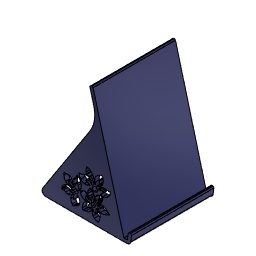
Portafoto (Autodesk Fusion 360 design; units mm, degrees)
Autodesk Fusion 360 part; units mm, degrees
sketch "Schizzo1" plane through (0, 0, 0) normal (0, 1, 0) x (1, 0, 0)
  line L0 (0, 0) -> (131.7113, 0) construction
  line L1 (79.5451, 0) -> (58.8396, -77.2741)
  line L2 (79.5451, 0) -> (81.9451, 0)
  line L3 (81.9451, 0) -> (82.641, -4.9513)
  line L4 (77.857, 2.2) -> (56.7146, -76.7047)
  line L5 (77.857, 2.2) -> (83.8576, 2.2)
  line L6 (83.8576, 2.2) -> (84.8196, -4.6452)
  line L7 (82.641, -4.9513) -> (84.8196, -4.6452)
  line L8 (77.857, 2.2) -> (22.857, 2.2)
  line L9 (22.857, 2.2) -> (61.7467, -57.9244)
  line L10 (56.7146, -76.7047) -> (58.8396, -77.2741)
  dimension "d1" = 75
  dimension "d2" = 2.4
  dimension "d3" = 5
  dimension "d4" = 80
  dimension "d5" = 2.2
  dimension "d6" = 55
  dimension "d23" = 98
  constraint coincident L0.start origin
  constraint horizontal L0
  constraint coincident L0 L1.start
  constraint coincident L0 L2.end
  constraint parallel L5 L8
  constraint coincident L4 L9.end
  measures "d1" angle of L0 L1
  measures "d2" distance of L1.start L2.end
  measures "d3" distance of L2.end L3.end
  measures "d4" distance of L1.start L1.end
  measures "d6" distance of L4.start L8.end
  measures "d23" angle of L2 L3
extrude "Estrusione1" add sketch "Schizzo1" along normal blind 55 contours L1 L2 L3 L4 L5 L6 L7 L10
extrude "Estrusione2" add sketch "Schizzo1" along normal blind 3 contours L4 L8 L9
fillet "Raccordo1" radius 2.5 1 edges at (83.8576, 27.5, -2.2)
fillet "Raccordo3" radius 0.75 2 edges at (82.641, 27.5, 4.9513) (84.8196, 27.5, 4.6452)
fillet "Raccordo4" radius 0.75 2 edges at (58.8396, 27.5, 77.2741) (56.7146, 27.5, 76.7047)
fillet "Raccordo5" radius 20 1 edges at (61.7467, 1.5, 57.9244)
fillet "Raccordo6" radius 2.5 1 edges at (22.857, 1.5, -2.2)
sketch "Schizzo3" plane through (0, 0, 0) normal (0, -1, 0) x (1, 0, 0)
  arc A0 (25.3523, 1.6578) -> (27.4515, -2.2) centre (27.4515, 0.3) ccw
  line L0 (27.4515, -2.2) -> (81.6844, -2.2)
  arc A1 (81.6844, -2.2) -> (84.16, -0.0479) centre (81.6844, 0.3) ccw
  line L1 (84.16, -0.0479) -> (84.7152, 3.9025)
  arc A2 (84.7152, 3.9025) -> (84.0769, 4.7495) centre (83.9725, 4.0068) ccw
  line L2 (84.0769, 4.7495) -> (83.3837, 4.847)
  arc A3 (83.3837, 4.847) -> (82.5366, 4.2086) centre (83.2793, 4.1043) ccw
  line L3 (82.5366, 4.2086) -> (81.9451, 0)
  line L4 (81.9451, 0) -> (79.5451, 0)
  line L5 (79.5451, 0) -> (59.0337, 76.5496)
  arc A4 (59.0337, 76.5496) -> (58.1152, 77.08) centre (58.3093, 76.3555) ccw
  line L6 (58.1152, 77.08) -> (57.439, 76.8988)
  arc A5 (57.439, 76.8988) -> (56.9087, 75.9802) centre (57.6331, 76.1743) ccw
  line L7 (56.9087, 75.9802) -> (59.4477, 66.5045)
  arc A6 (56.9224, 50.4659) -> (59.4477, 66.5045) centre (40.1292, 61.3281) ccw
  line L8 (56.9224, 50.4659) -> (25.3523, 1.6578)
  spline S0 degree 3 poles (64.7057, 28.6744) (64.5776, 28.5377) (64.293, 28.3413) (64.088, 28.2503) knots 0 0 0 0 1 1 1 1
  spline S1 degree 3 poles (64.088, 28.2503) (63.9912, 28.2076) (63.7037, 28.1022) (63.4533, 28.0197) knots 0 0 0 0 1 1 1 1
  spline S2 degree 3 poles (63.4533, 28.0197) (62.9096, 27.8432) (62.1667, 27.4931) (61.8422, 27.2625) knots 0 0 0 0 1 1 1 1
  spline S3 degree 3 poles (61.8422, 27.2625) (61.3212, 26.8953) (60.9512, 26.4627) (60.6609, 25.8706) knots 0 0 0 0 1 1 1 1
  spline S4 degree 3 poles (60.6609, 25.8706) (60.1001, 24.7377) (60.0005, 23.6077) (60.3392, 22.2271) knots 0 0 0 0 1 1 1 1
  spline S5 degree 3 poles (60.3392, 22.2271) (60.4104, 21.9453) (60.5897, 21.3817) (60.6239, 21.3476) knots 0 0 0 0 1 1 1 1
  spline S6 degree 3 poles (60.6239, 21.3476) (60.6381, 21.3305) (60.6495, 21.3874) (60.6495, 21.4785) knots 0 0 0 0 1 1 1 1
  spline S7 degree 3 poles (60.6495, 21.4785) (60.6495, 21.5696) (60.6694, 21.7859) (60.6922, 21.9624) knots 0 0 0 0 1 1 1 1
  spline S8 degree 3 poles (60.6922, 21.9624) (60.8317, 23.027) (61.2985, 23.8268) (62.0499, 24.288) knots 0 0 0 0 1 1 1 1
  spline S9 degree 3 poles (62.0499, 24.288) (62.3061, 24.4474) (62.7701, 24.6125) (62.9181, 24.5982) knots 0 0 0 0 1 1 1 1
  spline S10 degree 3 poles (62.9181, 24.5982) (63.0092, 24.5897) (63.0263, 24.5755) (63.0576, 24.4815) knots 0 0 0 0 1 1 1 1
  spline S11 degree 3 poles (63.0576, 24.4815) (63.2085, 24.0432) (63.1658, 23.3287) (62.9494, 22.7309) knots 0 0 0 0 1 1 1 1
  spline S12 degree 3 poles (62.9494, 22.7309) (62.7957, 22.3068) (62.6306, 22.1019) (61.808, 21.302) knots 0 0 0 0 1 1 1 1
  spline S13 degree 3 poles (61.808, 21.302) (61.5205, 21.0259) (61.3412, 20.7868) (61.2899, 20.6217) knots 0 0 0 0 1 1 1 1
  spline S14 degree 3 poles (61.2899, 20.6217) (61.27, 20.5591) (61.2757, 20.5562) (61.3497, 20.5733) knots 0 0 0 0 1 1 1 1
  spline S15 degree 3 poles (61.3497, 20.5733) (61.5461, 20.6189) (61.9987, 20.7783) (62.3004, 20.9092) knots 0 0 0 0 1 1 1 1
  spline S16 degree 3 poles (62.3004, 20.9092) (63.6354, 21.4813) (64.7142, 22.4121) (65.2579, 23.4653) knots 0 0 0 0 1 1 1 1
  spline S17 degree 3 poles (65.2579, 23.4653) (65.645, 24.2168) (65.8187, 25.0594) (65.7931, 26.0414) knots 0 0 0 0 1 1 1 1
  spline S18 degree 3 poles (65.7931, 26.0414) (65.776, 26.6135) (65.7304, 26.9039) (65.5853, 27.3735) knots 0 0 0 0 1 1 1 1
  spline S19 degree 3 poles (65.5853, 27.3735) (65.4515, 27.8005) (65.1498, 28.3556) (64.885, 28.6545) knots 0 0 0 0 1 1 1 1
  line L9 (64.885, 28.6545) -> (64.7911, 28.7655)
  line L10 (64.7911, 28.7655) -> (64.7057, 28.6744)
  spline S20 degree 3 poles (54.6121, 28.7114) (54.6093, 28.7) (54.6093, 28.6772) (54.6121, 28.663) knots 0 0 0 0 1 1 1 1
  spline S21 degree 3 poles (54.6121, 28.663) (54.6263, 28.5947) (54.5466, 27.9428) (54.4584, 27.4077) knots 0 0 0 0 1 1 1 1
  spline S22 degree 3 poles (54.4584, 27.4077) (54.3161, 26.5538) (54.2734, 26.1325) (54.2734, 25.6287) knots 0 0 0 0 1 1 1 1
  spline S23 degree 3 poles (54.2734, 25.6287) (54.2734, 25.1419) (54.3246, 24.7605) (54.4242, 24.4644) knots 0 0 0 0 1 1 1 1
  line L11 (54.4242, 24.4644) -> (54.4897, 24.2766)
  line L12 (54.4897, 24.2766) -> (54.8284, 24.2567)
  spline S24 degree 3 poles (54.8284, 24.2567) (55.3778, 24.2253) (55.8304, 24.0802) (56.2631, 23.7955) knots 0 0 0 0 1 1 1 1
  line L13 (56.2631, 23.7955) -> (56.4908, 23.6447)
  line L14 (56.4908, 23.6447) -> (56.5392, 23.8012)
  spline S25 degree 3 poles (56.5392, 23.8012) (56.5619, 23.8895) (56.6217, 24.0147) (56.6701, 24.0802) knots 0 0 0 0 1 1 1 1
  spline S26 degree 3 poles (56.6701, 24.0802) (56.7783, 24.2339) (57.043, 24.4616) (57.1113, 24.4616) knots 0 0 0 0 1 1 1 1
  spline S27 degree 3 poles (57.1113, 24.4616) (57.1398, 24.4616) (57.2508, 24.4303) (57.359, 24.3904) knots 0 0 0 0 1 1 1 1
  spline S28 degree 3 poles (57.359, 24.3904) (58.1901, 24.0972) (58.9331, 22.99) (59.4113, 21.3305) knots 0 0 0 0 1 1 1 1
  spline S29 degree 3 poles (59.4113, 21.3305) (59.4625, 21.1483) (59.5137, 20.9547) (59.5251, 20.895) knots 0 0 0 0 1 1 1 1
  spline S30 degree 3 poles (59.5251, 20.895) (59.5536, 20.7413) (59.5821, 20.7441) (59.6333, 20.912) knots 0 0 0 0 1 1 1 1
  spline S31 degree 3 poles (59.6333, 20.912) (59.9635, 21.9595) (59.8325, 23.6048) (59.3173, 24.917) knots 0 0 0 0 1 1 1 1
  spline S32 degree 3 poles (59.3173, 24.917) (58.8761, 26.0442) (58.3353, 26.827) (57.5127, 27.5386) knots 0 0 0 0 1 1 1 1
  spline S33 degree 3 poles (57.5127, 27.5386) (56.8437, 28.1136) (55.9101, 28.5377) (55.0135, 28.6715) knots 0 0 0 0 1 1 1 1
  spline S34 degree 3 poles (55.0135, 28.6715) (54.8968, 28.6915) (54.7573, 28.7114) (54.7089, 28.7199) knots 0 0 0 0 1 1 1 1
  spline S35 degree 3 poles (54.7089, 28.7199) (54.6577, 28.7285) (54.6121, 28.7228) (54.6121, 28.7114) knots 0 0 0 0 1 1 1 1
  spline S36 degree 3 poles (54.1026, 23.7614) (53.5646, 23.6874) (53.1206, 23.545) (52.2524, 23.1608) knots 0 0 0 0 1 1 1 1
  spline S37 degree 3 poles (52.2524, 23.1608) (51.333, 22.7537) (51.0284, 22.6569) (50.5018, 22.6114) knots 0 0 0 0 1 1 1 1
  spline S38 degree 3 poles (50.5018, 22.6114) (50.2314, 22.5886) (49.8073, 22.6085) (49.6165, 22.6569) knots 0 0 0 0 1 1 1 1
  spline S39 degree 3 poles (49.6165, 22.6569) (49.5482, 22.674) (49.5482, 22.6712) (49.5482, 22.489) knots 0 0 0 0 1 1 1 1
  spline S40 degree 3 poles (49.5482, 22.489) (49.5482, 21.7005) (50.035, 20.5648) (50.7324, 19.7393) knots 0 0 0 0 1 1 1 1
  spline S41 degree 3 poles (50.7324, 19.7393) (51.4326, 18.9024) (52.1755, 18.4385) (53.112, 18.2449) knots 0 0 0 0 1 1 1 1
  spline S42 degree 3 poles (53.112, 18.2449) (53.9375, 18.0741) (54.5409, 18.1424) (55.4604, 18.5096) knots 0 0 0 0 1 1 1 1
  spline S43 degree 3 poles (55.4604, 18.5096) (56.1094, 18.7687) (56.2204, 18.8) (56.5449, 18.817) knots 0 0 0 0 1 1 1 1
  spline S44 degree 3 poles (56.5449, 18.817) (56.8779, 18.837) (56.8807, 18.837) (56.764, 19.0732) knots 0 0 0 0 1 1 1 1
  spline S45 degree 3 poles (56.764, 19.0732) (56.5534, 19.4945) (55.9386, 19.8959) (55.1643, 20.1179) knots 0 0 0 0 1 1 1 1
  spline S46 degree 3 poles (55.1643, 20.1179) (54.8, 20.2232) (54.3189, 20.3057) (54.0741, 20.3057) knots 0 0 0 0 1 1 1 1
  spline S47 degree 3 poles (54.0741, 20.3057) (53.9261, 20.3057) (53.9261, 20.3057) (53.9432, 20.3854) knots 0 0 0 0 1 1 1 1
  spline S48 degree 3 poles (53.9432, 20.3854) (53.9546, 20.4281) (54.0087, 20.5278) (54.0627, 20.6075) knots 0 0 0 0 1 1 1 1
  spline S49 degree 3 poles (54.0627, 20.6075) (54.336, 21.0088) (54.9309, 21.2906) (55.6682, 21.3646) knots 0 0 0 0 1 1 1 1
  spline S50 degree 3 poles (55.6682, 21.3646) (55.9585, 21.3931) (56.0297, 21.3903) (56.2517, 21.3476) knots 0 0 0 0 1 1 1 1
  spline S51 degree 3 poles (56.2517, 21.3476) (56.7783, 21.2422) (57.1227, 21.0629) (57.5212, 20.6843) knots 0 0 0 0 1 1 1 1
  spline S52 degree 3 poles (57.5212, 20.6843) (57.7375, 20.4765) (58.099, 20.0382) (58.2186, 19.8332) knots 0 0 0 0 1 1 1 1
  spline S53 degree 3 poles (58.2186, 19.8332) (58.2812, 19.7308) (58.3011, 19.8275) (58.2983, 20.1862) knots 0 0 0 0 1 1 1 1
  spline S54 degree 3 poles (58.2983, 20.1862) (58.2954, 20.5875) (58.23, 20.9377) (58.082, 21.3561) knots 0 0 0 0 1 1 1 1
  spline S55 degree 3 poles (58.082, 21.3561) (57.6521, 22.5772) (56.6559, 23.4539) (55.412, 23.7073) knots 0 0 0 0 1 1 1 1
  spline S56 degree 3 poles (55.412, 23.7073) (55.2013, 23.7528) (54.3047, 23.787) (54.1026, 23.7614) knots 0 0 0 0 1 1 1 1
  spline S57 degree 3 poles (65.8443, 22.1673) (65.7988, 22.1616) (65.6621, 22.1417) (65.5454, 22.1246) knots 0 0 0 0 1 1 1 1
  spline S58 degree 3 poles (65.5454, 22.1246) (65.0444, 22.0563) (64.3328, 21.7574) (63.9201, 21.4472) knots 0 0 0 0 1 1 1 1
  spline S59 degree 3 poles (63.9201, 21.4472) (63.5273, 21.1483) (63.0918, 20.6132) (62.9124, 20.209) knots 0 0 0 0 1 1 1 1
  spline S60 degree 3 poles (62.9124, 20.209) (62.8185, 19.9983) (62.7103, 19.6482) (62.6676, 19.4319) knots 0 0 0 0 1 1 1 1
  spline S61 degree 3 poles (62.6676, 19.4319) (62.6392, 19.2839) (62.642, 19.2355) (62.6847, 19.1045) knots 0 0 0 0 1 1 1 1
  spline S62 degree 3 poles (62.6847, 19.1045) (62.7559, 18.891) (62.7559, 18.891) (62.8413, 19.0277) knots 0 0 0 0 1 1 1 1
  spline S63 degree 3 poles (62.8413, 19.0277) (62.9523, 19.2042) (63.1743, 19.4205) (63.3622, 19.5344) knots 0 0 0 0 1 1 1 1
  spline S64 degree 3 poles (63.3622, 19.5344) (63.7208, 19.7478) (64.3072, 19.8759) (64.7484, 19.8389) knots 0 0 0 0 1 1 1 1
  spline S65 degree 3 poles (64.7484, 19.8389) (64.9647, 19.819) (65.4031, 19.7251) (65.497, 19.6767) knots 0 0 0 0 1 1 1 1
  spline S66 degree 3 poles (65.497, 19.6767) (65.5995, 19.6197) (65.5113, 19.1472) (65.3291, 18.7857) knots 0 0 0 0 1 1 1 1
  spline S67 degree 3 poles (65.3291, 18.7857) (65.0444, 18.2278) (64.4552, 17.6187) (63.9002, 17.3113) knots 0 0 0 0 1 1 1 1
  line L15 (63.9002, 17.3113) -> (63.7237, 17.2116)
  line L16 (63.7237, 17.2116) -> (63.9571, 17.1376)
  spline S68 degree 3 poles (63.9571, 17.1376) (64.5805, 16.9412) (64.9533, 16.8843) (65.5739, 16.8843) knots 0 0 0 0 1 1 1 1
  spline S69 degree 3 poles (65.5739, 16.8843) (66.3396, 16.8871) (66.9459, 17.0323) (67.666, 17.391) knots 0 0 0 0 1 1 1 1
  spline S70 degree 3 poles (67.666, 17.391) (68.1357, 17.6215) (68.4887, 17.8749) (68.9014, 18.2705) knots 0 0 0 0 1 1 1 1
  spline S71 degree 3 poles (68.9014, 18.2705) (69.6557, 18.9992) (70.1681, 19.8617) (70.373, 20.7555) knots 0 0 0 0 1 1 1 1
  spline S72 degree 3 poles (70.373, 20.7555) (70.447, 21.0828) (70.4897, 21.6322) (70.4584, 21.8485) knots 0 0 0 0 1 1 1 1
  line L17 (70.4584, 21.8485) -> (70.4385, 21.9795)
  line L18 (70.4385, 21.9795) -> (70.3161, 21.9282)
  spline S73 degree 3 poles (70.3161, 21.9282) (70.0058, 21.7888) (69.4622, 21.8001) (68.2866, 21.9681) knots 0 0 0 0 1 1 1 1
  spline S74 degree 3 poles (68.2866, 21.9681) (67.9137, 22.0222) (67.4355, 22.0876) (67.2248, 22.1104) knots 0 0 0 0 1 1 1 1
  spline S75 degree 3 poles (67.2248, 22.1104) (66.8349, 22.156) (66.0009, 22.1901) (65.8443, 22.1673) knots 0 0 0 0 1 1 1 1
  spline S76 degree 3 poles (48.2844, 20.7099) (48.2759, 20.7014) (48.2673, 20.6502) (48.2673, 20.5932) knots 0 0 0 0 1 1 1 1
  spline S77 degree 3 poles (48.2673, 20.5932) (48.2673, 20.3655) (48.0937, 19.9841) (47.8233, 19.6027) knots 0 0 0 0 1 1 1 1
  spline S78 degree 3 poles (47.8233, 19.6027) (47.7293, 19.4746) (47.4561, 19.1387) (47.2141, 18.854) knots 0 0 0 0 1 1 1 1
  spline S79 degree 3 poles (47.2141, 18.854) (46.2805, 17.7582) (45.9218, 17.2059) (45.6913, 16.5114) knots 0 0 0 0 1 1 1 1
  spline S80 degree 3 poles (45.6913, 16.5114) (45.4066, 15.6432) (45.4493, 14.5587) (45.7994, 13.8443) knots 0 0 0 0 1 1 1 1
  spline S81 degree 3 poles (45.7994, 13.8443) (45.9617, 13.5084) (46.3061, 13.1611) (46.6221, 13.0102) knots 0 0 0 0 1 1 1 1
  spline S82 degree 3 poles (46.6221, 13.0102) (46.7445, 12.9505) (46.8839, 12.8964) (46.9323, 12.885) knots 0 0 0 0 1 1 1 1
  line L19 (46.9323, 12.885) -> (47.0206, 12.8679)
  line L20 (47.0206, 12.8679) -> (46.9949, 13.0074)
  spline S83 degree 3 poles (46.9949, 13.0074) (46.9551, 13.2436) (46.9722, 13.8955) (47.0234, 14.1061) knots 0 0 0 0 1 1 1 1
  spline S84 degree 3 poles (47.0234, 14.1061) (47.1003, 14.4135) (47.234, 14.7352) (47.3906, 14.9743) knots 0 0 0 0 1 1 1 1
  spline S85 degree 3 poles (47.3906, 14.9743) (47.5699, 15.2504) (47.9684, 15.6489) (48.2018, 15.7912) knots 0 0 0 0 1 1 1 1
  line L21 (48.2018, 15.7912) -> (48.3812, 15.8966)
  line L22 (48.3812, 15.8966) -> (48.4979, 15.8026)
  spline S86 degree 3 poles (48.4979, 15.8026) (48.6459, 15.6831) (48.8452, 15.4184) (48.9647, 15.1821) knots 0 0 0 0 1 1 1 1
  spline S87 degree 3 poles (48.9647, 15.1821) (49.2636, 14.5843) (49.386, 13.9012) (49.3888, 12.8138) knots 0 0 0 0 1 1 1 1
  line L23 (49.3888, 12.8138) -> (49.3888, 12.199)
  line L24 (49.3888, 12.199) -> (49.5454, 12.2986)
  spline S88 degree 3 poles (49.5454, 12.2986) (50.2912, 12.7711) (50.7836, 13.4714) (51.0142, 14.3822) knots 0 0 0 0 1 1 1 1
  spline S89 degree 3 poles (51.0142, 14.3822) (51.2277, 15.2305) (51.2163, 16.3292) (50.9857, 17.3027) knots 0 0 0 0 1 1 1 1
  spline S90 degree 3 poles (50.9857, 17.3027) (50.6612, 18.669) (49.867, 19.8218) (48.8081, 20.468) knots 0 0 0 0 1 1 1 1
  spline S91 degree 3 poles (48.8081, 20.468) (48.5833, 20.6046) (48.3072, 20.7327) (48.2844, 20.7099) knots 0 0 0 0 1 1 1 1
  spline S92 degree 3 poles (59.9521, 20.0809) (59.1038, 19.9414) (58.5146, 19.2981) (58.5146, 18.5125) knots 0 0 0 0 1 1 1 1
  spline S93 degree 3 poles (58.5146, 18.5125) (58.5146, 17.8179) (58.9786, 17.2287) (59.7101, 16.9953) knots 0 0 0 0 1 1 1 1
  spline S94 degree 3 poles (59.7101, 16.9953) (59.9606, 16.9156) (60.473, 16.9099) (60.7206, 16.9868) knots 0 0 0 0 1 1 1 1
  spline S95 degree 3 poles (60.7206, 16.9868) (61.2871, 17.1575) (61.7169, 17.5589) (61.8905, 18.0855) knots 0 0 0 0 1 1 1 1
  spline S96 degree 3 poles (61.8905, 18.0855) (61.9617, 18.299) (61.9617, 18.726) (61.8905, 18.9394) knots 0 0 0 0 1 1 1 1
  spline S97 degree 3 poles (61.8905, 18.9394) (61.7169, 19.4689) (61.2871, 19.8702) (60.732, 20.0325) knots 0 0 0 0 1 1 1 1
  spline S98 degree 3 poles (60.732, 20.0325) (60.5385, 20.0866) (60.1457, 20.1122) (59.9521, 20.0809) knots 0 0 0 0 1 1 1 1
  spline S99 degree 3 poles (41.1483, 18.0143) (41.1369, 18.0058) (40.7839, 17.9916) (40.3655, 17.9859) knots 0 0 0 0 1 1 1 1
  line L25 (40.3655, 17.9859) -> (39.5998, 17.9773)
  line L26 (39.5998, 17.9773) -> (39.5656, 17.7809)
  spline S100 degree 3 poles (39.5656, 17.7809) (39.5087, 17.4707) (39.4888, 16.6907) (39.5258, 16.3065) knots 0 0 0 0 1 1 1 1
  spline S101 degree 3 poles (39.5258, 16.3065) (39.6397, 15.1451) (40.0524, 14.0663) (40.69, 13.2636) knots 0 0 0 0 1 1 1 1
  spline S102 degree 3 poles (40.69, 13.2636) (41.1397, 12.7) (41.4358, 12.4893) (42.0962, 12.2673) knots 0 0 0 0 1 1 1 1
  spline S103 degree 3 poles (42.0962, 12.2673) (42.822, 12.0254) (43.8069, 11.92) (44.6665, 11.9912) knots 0 0 0 0 1 1 1 1
  spline S104 degree 3 poles (44.6665, 11.9912) (45.2387, 12.0396) (45.7624, 12.1648) (45.7624, 12.2502) knots 0 0 0 0 1 1 1 1
  spline S105 degree 3 poles (45.7624, 12.2502) (45.7624, 12.3128) (45.5119, 12.3897) (44.9369, 12.5036) knots 0 0 0 0 1 1 1 1
  spline S106 degree 3 poles (44.9369, 12.5036) (44.2965, 12.6317) (44.0118, 12.7085) (43.6703, 12.848) knots 0 0 0 0 1 1 1 1
  spline S107 degree 3 poles (43.6703, 12.848) (43.0469, 13.1042) (42.6171, 13.4998) (42.4093, 14.0065) knots 0 0 0 0 1 1 1 1
  line L27 (42.4093, 14.0065) -> (42.3495, 14.1574)
  line L28 (42.3495, 14.1574) -> (42.4207, 14.2399)
  spline S108 degree 3 poles (42.4207, 14.2399) (42.6939, 14.5644) (43.6503, 14.6526) (44.2879, 14.4135) knots 0 0 0 0 1 1 1 1
  spline S109 degree 3 poles (44.2879, 14.4135) (44.6836, 14.2655) (45.0793, 13.9581) (45.3013, 13.6251) knots 0 0 0 0 1 1 1 1
  spline S110 degree 3 poles (45.3013, 13.6251) (45.3554, 13.5425) (45.4066, 13.4742) (45.4152, 13.4742) knots 0 0 0 0 1 1 1 1
  spline S111 degree 3 poles (45.4152, 13.4742) (45.4237, 13.4742) (45.4208, 13.7219) (45.4123, 14.0236) knots 0 0 0 0 1 1 1 1
  spline S112 degree 3 poles (45.4123, 14.0236) (45.3924, 14.738) (45.2899, 15.35) (45.0907, 15.9364) knots 0 0 0 0 1 1 1 1
  spline S113 degree 3 poles (45.0907, 15.9364) (44.7605, 16.9127) (44.1769, 17.5731) (43.4112, 17.8407) knots 0 0 0 0 1 1 1 1
  spline S114 degree 3 poles (43.4112, 17.8407) (42.9928, 17.9887) (42.8362, 18.0058) (41.9766, 18.02) knots 0 0 0 0 1 1 1 1
  spline S115 degree 3 poles (41.9766, 18.02) (41.5297, 18.0286) (41.1568, 18.0257) (41.1483, 18.0143) knots 0 0 0 0 1 1 1 1
  spline S116 degree 3 poles (56.9149, 17.539) (56.8751, 17.4564) (56.7327, 17.2543) (56.5961, 17.0892) knots 0 0 0 0 1 1 1 1
  spline S117 degree 3 poles (56.5961, 17.0892) (56.0211, 16.4004) (55.7592, 15.8766) (55.5486, 15.0142) knots 0 0 0 0 1 1 1 1
  spline S118 degree 3 poles (55.5486, 15.0142) (55.4746, 14.7039) (55.449, 14.0834) (55.4974, 13.756) knots 0 0 0 0 1 1 1 1
  spline S119 degree 3 poles (55.4974, 13.756) (55.5628, 13.2977) (55.7678, 12.7142) (56.0154, 12.2645) knots 0 0 0 0 1 1 1 1
  spline S120 degree 3 poles (56.0154, 12.2645) (56.5107, 11.3764) (57.396, 10.5167) (57.9482, 10.3886) knots 0 0 0 0 1 1 1 1
  line L29 (57.9482, 10.3886) -> (58.025, 10.3716)
  line L30 (58.025, 10.3716) -> (57.9283, 10.5936)
  spline S121 degree 3 poles (57.9283, 10.5936) (57.5639, 11.4361) (57.5525, 12.4409) (57.8998, 13.033) knots 0 0 0 0 1 1 1 1
  spline S122 degree 3 poles (57.8998, 13.033) (57.9823, 13.1725) (58.0165, 13.1839) (58.1531, 13.1156) knots 0 0 0 0 1 1 1 1
  spline S123 degree 3 poles (58.1531, 13.1156) (58.5402, 12.9163) (58.99, 12.3698) (59.3003, 11.7236) knots 0 0 0 0 1 1 1 1
  spline S124 degree 3 poles (59.3003, 11.7236) (59.4454, 11.4247) (59.5963, 10.9408) (59.5963, 10.7758) knots 0 0 0 0 1 1 1 1
  spline S125 degree 3 poles (59.5963, 10.7758) (59.5963, 10.7188) (59.602, 10.7131) (59.639, 10.7416) knots 0 0 0 0 1 1 1 1
  spline S126 degree 3 poles (59.639, 10.7416) (59.7443, 10.8298) (59.9094, 11.476) (59.9692, 12.0424) knots 0 0 0 0 1 1 1 1
  spline S127 degree 3 poles (59.9692, 12.0424) (60.0147, 12.4836) (59.9891, 13.6507) (59.9236, 14.0577) knots 0 0 0 0 1 1 1 1
  spline S128 degree 3 poles (59.9236, 14.0577) (59.8354, 14.6156) (59.602, 15.1906) (59.212, 15.8083) knots 0 0 0 0 1 1 1 1
  spline S129 degree 3 poles (59.212, 15.8083) (58.805, 16.4488) (58.2613, 17.0209) (57.7603, 17.3397) knots 0 0 0 0 1 1 1 1
  spline S130 degree 3 poles (57.7603, 17.3397) (57.5952, 17.4422) (57.1682, 17.6443) (57.0601, 17.6728) knots 0 0 0 0 1 1 1 1
  spline S131 degree 3 poles (57.0601, 17.6728) (56.9889, 17.6898) (56.9775, 17.6785) (56.9149, 17.539) knots 0 0 0 0 1 1 1 1
  spline S132 degree 3 poles (63.2825, 16.4203) (62.3403, 16.2666) (61.5376, 15.8083) (61.0394, 15.1394) knots 0 0 0 0 1 1 1 1
  spline S133 degree 3 poles (61.0394, 15.1394) (60.843, 14.8804) (60.6352, 14.4619) (60.5072, 14.0777) knots 0 0 0 0 1 1 1 1
  spline S134 degree 3 poles (60.5072, 14.0777) (60.2282, 13.2465) (60.1798, 12.2104) (60.3791, 11.439) knots 0 0 0 0 1 1 1 1
  spline S135 degree 3 poles (60.3791, 11.439) (60.4445, 11.1856) (60.6153, 10.7957) (60.6723, 10.7587) knots 0 0 0 0 1 1 1 1
  spline S136 degree 3 poles (60.6723, 10.7587) (60.6865, 10.7501) (60.7064, 10.8555) (60.7178, 10.9921) knots 0 0 0 0 1 1 1 1
  spline S137 degree 3 poles (60.7178, 10.9921) (60.8117, 12.1904) (61.3127, 12.9248) (62.1809, 13.1469) knots 0 0 0 0 1 1 1 1
  spline S138 degree 3 poles (62.1809, 13.1469) (62.4399, 13.2152) (62.4798, 13.2009) (62.5082, 13.0472) knots 0 0 0 0 1 1 1 1
  spline S139 degree 3 poles (62.5082, 13.0472) (62.5424, 12.8679) (62.5111, 12.552) (62.4456, 12.3555) knots 0 0 0 0 1 1 1 1
  spline S140 degree 3 poles (62.4456, 12.3555) (62.3574, 12.1022) (62.2435, 11.9286) (61.9275, 11.5528) knots 0 0 0 0 1 1 1 1
  spline S141 degree 3 poles (61.9275, 11.5528) (61.4522, 10.9892) (61.3156, 10.7473) (61.2842, 10.4029) knots 0 0 0 0 1 1 1 1
  line L31 (61.2842, 10.4029) -> (61.2672, 10.215)
  line L32 (61.2672, 10.215) -> (61.4493, 10.3829)
  spline S142 degree 3 poles (61.4493, 10.3829) (61.734, 10.642) (62.0642, 10.8469) (62.7559, 11.1942) knots 0 0 0 0 1 1 1 1
  spline S143 degree 3 poles (62.7559, 11.1942) (63.1088, 11.3707) (63.5045, 11.5898) (63.6383, 11.6752) knots 0 0 0 0 1 1 1 1
  spline S144 degree 3 poles (63.6383, 11.6752) (64.3897, 12.1677) (65.0017, 13.144) (65.2608, 14.2598) knots 0 0 0 0 1 1 1 1
  spline S145 degree 3 poles (65.2608, 14.2598) (65.2921, 14.3879) (65.3547, 14.7665) (65.4031, 15.0967) knots 0 0 0 0 1 1 1 1
  spline S146 degree 3 poles (65.4031, 15.0967) (65.4515, 15.4269) (65.517, 15.777) (65.5454, 15.8738) knots 0 0 0 0 1 1 1 1
  spline S147 degree 3 poles (65.5454, 15.8738) (65.5767, 15.9706) (65.6023, 16.0645) (65.6023, 16.0816) knots 0 0 0 0 1 1 1 1
  spline S148 degree 3 poles (65.6023, 16.0816) (65.6023, 16.1186) (65.3376, 16.241) (65.1184, 16.3008) knots 0 0 0 0 1 1 1 1
  spline S149 degree 3 poles (65.1184, 16.3008) (64.5975, 16.4459) (63.7778, 16.5) (63.2825, 16.4203) knots 0 0 0 0 1 1 1 1
  spline S150 degree 3 poles (53.3056, 13.9268) (52.8473, 13.8699) (52.352, 13.6735) (51.6689, 13.2806) knots 0 0 0 0 1 1 1 1
  spline S151 degree 3 poles (51.6689, 13.2806) (51.1593, 12.9875) (50.8633, 12.8594) (50.5843, 12.8224) knots 0 0 0 0 1 1 1 1
  spline S152 degree 3 poles (50.5843, 12.8224) (50.4819, 12.8053) (50.3908, 12.7882) (50.3822, 12.7797) knots 0 0 0 0 1 1 1 1
  spline S153 degree 3 poles (50.3822, 12.7797) (50.3509, 12.7512) (50.5217, 11.9997) (50.6299, 11.6724) knots 0 0 0 0 1 1 1 1
  spline S154 degree 3 poles (50.6299, 11.6724) (51.1024, 10.2605) (52.0304, 9.2956) (53.3198, 8.88) knots 0 0 0 0 1 1 1 1
  spline S155 degree 3 poles (53.3198, 8.88) (54.2136, 8.5925) (55.3664, 8.6153) (56.2374, 8.9398) knots 0 0 0 0 1 1 1 1
  spline S156 degree 3 poles (56.2374, 8.9398) (56.6445, 9.0906) (56.6388, 9.0849) (56.505, 9.1646) knots 0 0 0 0 1 1 1 1
  spline S157 degree 3 poles (56.505, 9.1646) (56.3399, 9.2643) (56.0211, 9.3611) (55.5258, 9.4635) knots 0 0 0 0 1 1 1 1
  spline S158 degree 3 poles (55.5258, 9.4635) (54.7203, 9.6286) (54.4271, 9.7738) (54.1396, 10.1581) knots 0 0 0 0 1 1 1 1
  spline S159 degree 3 poles (54.1396, 10.1581) (53.9574, 10.4) (53.7325, 10.8725) (53.7325, 11.012) knots 0 0 0 0 1 1 1 1
  spline S160 degree 3 poles (53.7325, 11.012) (53.7325, 11.049) (54.0257, 11.1913) (54.2734, 11.2739) knots 0 0 0 0 1 1 1 1
  spline S161 degree 3 poles (54.2734, 11.2739) (54.3815, 11.3109) (54.5153, 11.3251) (54.7146, 11.3251) knots 0 0 0 0 1 1 1 1
  spline S162 degree 3 poles (54.7146, 11.3251) (54.9736, 11.3251) (55.0135, 11.3166) (55.1672, 11.2397) knots 0 0 0 0 1 1 1 1
  spline S163 degree 3 poles (55.1672, 11.2397) (55.3835, 11.1316) (55.5941, 10.8953) (55.7877, 10.5423) knots 0 0 0 0 1 1 1 1
  line L33 (55.7877, 10.5423) -> (55.9386, 10.2719)
  line L34 (55.9386, 10.2719) -> (55.9898, 10.4854)
  spline S164 degree 3 poles (55.9898, 10.4854) (56.0638, 10.7758) (56.0667, 11.2995) (55.9983, 11.624) knots 0 0 0 0 1 1 1 1
  spline S165 degree 3 poles (55.9983, 11.624) (55.6909, 13.0814) (54.5182, 14.0834) (53.3056, 13.9268) knots 0 0 0 0 1 1 1 1
  spline S166 degree 3 poles (47.1999, 12.2246) (46.6904, 12.0794) (46.2776, 11.6553) (46.1894, 11.1942) knots 0 0 0 0 1 1 1 1
  spline S167 degree 3 poles (46.1894, 11.1942) (46.104, 10.7473) (46.2292, 10.3602) (46.5651, 10.0243) knots 0 0 0 0 1 1 1 1
  spline S168 degree 3 poles (46.5651, 10.0243) (47.1088, 9.4806) (48.0624, 9.4664) (48.6402, 9.9958) knots 0 0 0 0 1 1 1 1
  spline S169 degree 3 poles (48.6402, 9.9958) (49.4258, 10.7188) (49.0672, 11.9542) (47.9912, 12.2331) knots 0 0 0 0 1 1 1 1
  spline S170 degree 3 poles (47.9912, 12.2331) (47.7692, 12.2929) (47.4162, 12.2872) (47.1999, 12.2246) knots 0 0 0 0 1 1 1 1
  spline S171 degree 3 poles (41.5496, 11.7521) (40.6701, 11.6098) (39.7621, 11.0889) (39.1358, 10.3716) knots 0 0 0 0 1 1 1 1
  spline S172 degree 3 poles (39.1358, 10.3716) (38.6206, 9.7823) (38.2534, 9.0337) (38.1054, 8.2765) knots 0 0 0 0 1 1 1 1
  spline S173 degree 3 poles (38.1054, 8.2765) (38.0485, 7.9834) (38.0001, 7.4681) (38.0286, 7.4681) knots 0 0 0 0 1 1 1 1
  spline S174 degree 3 poles (38.0286, 7.4681) (38.0371, 7.4681) (38.1509, 7.4938) (38.2819, 7.5251) knots 0 0 0 0 1 1 1 1
  spline S175 degree 3 poles (38.2819, 7.5251) (38.6235, 7.6105) (39.0305, 7.6276) (39.3465, 7.5706) knots 0 0 0 0 1 1 1 1
  spline S176 degree 3 poles (39.3465, 7.5706) (39.7051, 7.508) (39.9955, 7.4027) (40.6245, 7.1066) knots 0 0 0 0 1 1 1 1
  spline S177 degree 3 poles (40.6245, 7.1066) (41.5354, 6.6768) (41.8371, 6.5857) (42.3666, 6.5857) knots 0 0 0 0 1 1 1 1
  spline S178 degree 3 poles (42.3666, 6.5857) (43.3258, 6.5857) (44.416, 7.1607) (45.1333, 8.0517) knots 0 0 0 0 1 1 1 1
  spline S179 degree 3 poles (45.1333, 8.0517) (45.418, 8.4018) (45.8137, 9.0195) (45.7795, 9.0565) knots 0 0 0 0 1 1 1 1
  spline S180 degree 3 poles (45.7795, 9.0565) (45.771, 9.0622) (45.5746, 9.0963) (45.344, 9.1276) knots 0 0 0 0 1 1 1 1
  spline S181 degree 3 poles (45.344, 9.1276) (44.7462, 9.2102) (43.6162, 9.2102) (43.249, 9.1276) knots 0 0 0 0 1 1 1 1
  spline S182 degree 3 poles (43.249, 9.1276) (42.9672, 9.065) (42.9729, 9.0593) (43.1237, 9.2956) knots 0 0 0 0 1 1 1 1
  spline S183 degree 3 poles (43.1237, 9.2956) (43.3942, 9.7169) (43.7557, 9.973) (44.2965, 10.1353) knots 0 0 0 0 1 1 1 1
  spline S184 degree 3 poles (44.2965, 10.1353) (44.4303, 10.1751) (44.5669, 10.1865) (44.9455, 10.1865) knots 0 0 0 0 1 1 1 1
  line L35 (44.9455, 10.1865) -> (45.4265, 10.1865)
  line L36 (45.4265, 10.1865) -> (45.4095, 10.2719)
  spline S185 degree 3 poles (45.4095, 10.2719) (45.3582, 10.5253) (45.0878, 10.8868) (44.769, 11.1202) knots 0 0 0 0 1 1 1 1
  spline S186 degree 3 poles (44.769, 11.1202) (44.4559, 11.3536) (43.9293, 11.5699) (43.3572, 11.7009) knots 0 0 0 0 1 1 1 1
  spline S187 degree 3 poles (43.3572, 11.7009) (43.0867, 11.7606) (42.9615, 11.772) (42.4178, 11.7806) knots 0 0 0 0 1 1 1 1
  spline S188 degree 3 poles (42.4178, 11.7806) (41.9738, 11.7891) (41.7204, 11.7806) (41.5496, 11.7521) knots 0 0 0 0 1 1 1 1
  spline S189 degree 3 poles (64.3527, 11.5386) (63.2455, 11.3109) (62.2919, 10.642) (61.5063, 9.5404) knots 0 0 0 0 1 1 1 1
  spline S190 degree 3 poles (61.5063, 9.5404) (61.4408, 9.4521) (61.3896, 9.3724) (61.3896, 9.3639) knots 0 0 0 0 1 1 1 1
  spline S191 degree 3 poles (61.3896, 9.3639) (61.3896, 9.3554) (61.4693, 9.4009) (61.5632, 9.4664) knots 0 0 0 0 1 1 1 1
  spline S192 degree 3 poles (61.5632, 9.4664) (61.7966, 9.6201) (62.0386, 9.7282) (62.3317, 9.808) knots 0 0 0 0 1 1 1 1
  spline S193 degree 3 poles (62.3317, 9.808) (62.5253, 9.8592) (62.642, 9.8706) (62.9551, 9.8706) knots 0 0 0 0 1 1 1 1
  spline S194 degree 3 poles (62.9551, 9.8706) (63.3906, 9.8706) (63.6354, 9.8193) (63.9799, 9.6485) knots 0 0 0 0 1 1 1 1
  spline S195 degree 3 poles (63.9799, 9.6485) (64.1848, 9.5461) (64.4353, 9.3867) (64.4353, 9.3554) knots 0 0 0 0 1 1 1 1
  spline S196 degree 3 poles (64.4353, 9.3554) (64.4353, 9.2529) (63.9855, 8.8743) (63.718, 8.7491) knots 0 0 0 0 1 1 1 1
  spline S197 degree 3 poles (63.718, 8.7491) (63.4561, 8.6267) (63.2142, 8.584) (62.6079, 8.5498) knots 0 0 0 0 1 1 1 1
  spline S198 degree 3 poles (62.6079, 8.5498) (62.0499, 8.5213) (61.8735, 8.4957) (61.697, 8.416) knots 0 0 0 0 1 1 1 1
  spline S199 degree 3 poles (61.697, 8.416) (61.5888, 8.3705) (61.5774, 8.3221) (61.6742, 8.3221) knots 0 0 0 0 1 1 1 1
  spline S200 degree 3 poles (61.6742, 8.3221) (61.7568, 8.3221) (62.0129, 8.1314) (62.3801, 7.7983) knots 0 0 0 0 1 1 1 1
  spline S201 degree 3 poles (62.3801, 7.7983) (62.9779, 7.2575) (63.3707, 7.0127) (63.9485, 6.822) knots 0 0 0 0 1 1 1 1
  spline S202 degree 3 poles (63.9485, 6.822) (64.7569, 6.5573) (65.4572, 6.5829) (66.5417, 6.9188) knots 0 0 0 0 1 1 1 1
  spline S203 degree 3 poles (66.5417, 6.9188) (67.0569, 7.0753) (67.5066, 7.2689) (68.5627, 7.7813) knots 0 0 0 0 1 1 1 1
  spline S204 degree 3 poles (68.5627, 7.7813) (69.428, 8.2025) (69.8351, 8.379) (70.0258, 8.4132) knots 0 0 0 0 1 1 1 1
  spline S205 degree 3 poles (70.0258, 8.4132) (70.0656, 8.4189) (70.0087, 8.4673) (69.8265, 8.584) knots 0 0 0 0 1 1 1 1
  spline S206 degree 3 poles (69.8265, 8.584) (69.4679, 8.8117) (69.2344, 9.0138) (68.3862, 9.8307) knots 0 0 0 0 1 1 1 1
  spline S207 degree 3 poles (68.3862, 9.8307) (67.4298, 10.753) (67.017, 11.0632) (66.4022, 11.328) knots 0 0 0 0 1 1 1 1
  spline S208 degree 3 poles (66.4022, 11.328) (65.9695, 11.5158) (65.6764, 11.5728) (65.1184, 11.5842) knots 0 0 0 0 1 1 1 1
  spline S209 degree 3 poles (65.1184, 11.5842) (64.7114, 11.5927) (64.5719, 11.5842) (64.3527, 11.5386) knots 0 0 0 0 1 1 1 1
  spline S210 degree 3 poles (58.8989, 10.1695) (58.1987, 10.0841) (57.6578, 9.5062) (57.6578, 8.8515) knots 0 0 0 0 1 1 1 1
  spline S211 degree 3 poles (57.6578, 8.8515) (57.6578, 8.3933) (57.8912, 7.9862) (58.3068, 7.7243) knots 0 0 0 0 1 1 1 1
  spline S212 degree 3 poles (58.3068, 7.7243) (58.6, 7.5365) (59.1095, 7.4625) (59.4824, 7.5507) knots 0 0 0 0 1 1 1 1
  spline S213 degree 3 poles (59.4824, 7.5507) (59.8667, 7.6418) (60.2481, 7.9407) (60.4218, 8.2794) knots 0 0 0 0 1 1 1 1
  spline S214 degree 3 poles (60.4218, 8.2794) (60.9085, 9.2387) (60.046, 10.3118) (58.8989, 10.1695) knots 0 0 0 0 1 1 1 1
  spline S215 degree 3 poles (48.5861, 8.7946) (48.5548, 8.6637) (48.4865, 8.4587) (48.4381, 8.3392) knots 0 0 0 0 1 1 1 1
  spline S216 degree 3 poles (48.4381, 8.3392) (48.2559, 7.9037) (48.0766, 7.6845) (47.217, 6.8562) knots 0 0 0 0 1 1 1 1
  spline S217 degree 3 poles (47.217, 6.8562) (47.0405, 6.6825) (46.8384, 6.4804) (46.7729, 6.4007) knots 0 0 0 0 1 1 1 1
  spline S218 degree 3 poles (46.7729, 6.4007) (46.5993, 6.1958) (46.3459, 5.8172) (46.2292, 5.5809) knots 0 0 0 0 1 1 1 1
  line L37 (46.2292, 5.5809) -> (46.1268, 5.3788)
  line L38 (46.1268, 5.3788) -> (46.0556, 5.5468)
  spline S219 degree 3 poles (46.0556, 5.5468) (45.6685, 6.4605) (45.8649, 7.6759) (46.5082, 8.3648) knots 0 0 0 0 1 1 1 1
  spline S220 degree 3 poles (46.5082, 8.3648) (46.6761, 8.5441) (46.6961, 8.5783) (46.6448, 8.5783) knots 0 0 0 0 1 1 1 1
  spline S221 degree 3 poles (46.6448, 8.5783) (46.4342, 8.5783) (45.9133, 8.3392) (45.5888, 8.0944) knots 0 0 0 0 1 1 1 1
  spline S222 degree 3 poles (45.5888, 8.0944) (45.3411, 7.9094) (44.9882, 7.5336) (44.8089, 7.266) knots 0 0 0 0 1 1 1 1
  spline S223 degree 3 poles (44.8089, 7.266) (44.3847, 6.637) (44.1513, 5.8884) (44.12, 5.0629) knots 0 0 0 0 1 1 1 1
  spline S224 degree 3 poles (44.12, 5.0629) (44.0858, 4.1378) (44.2794, 3.5628) (45.0223, 2.373) knots 0 0 0 0 1 1 1 1
  spline S225 degree 3 poles (45.0223, 2.373) (45.2131, 2.0684) (45.4208, 1.724) (45.4835, 1.613) knots 0 0 0 0 1 1 1 1
  spline S226 degree 3 poles (45.4835, 1.613) (45.5461, 1.4991) (45.603, 1.4052) (45.6087, 1.4052) knots 0 0 0 0 1 1 1 1
  spline S227 degree 3 poles (45.6087, 1.4052) (45.6144, 1.4052) (45.6884, 1.4592) (45.771, 1.5276) knots 0 0 0 0 1 1 1 1
  spline S228 degree 3 poles (45.771, 1.5276) (46.0186, 1.7297) (46.3516, 1.9147) (47.3052, 2.3843) knots 0 0 0 0 1 1 1 1
  spline S229 degree 3 poles (47.3052, 2.3843) (48.7797, 3.1102) (49.2266, 3.4546) (49.6536, 4.2004) knots 0 0 0 0 1 1 1 1
  spline S230 degree 3 poles (49.6536, 4.2004) (50.1801, 5.1198) (50.2485, 6.4719) (49.8215, 7.5934) knots 0 0 0 0 1 1 1 1
  spline S231 degree 3 poles (49.8215, 7.5934) (49.6279, 8.1029) (49.238, 8.6324) (48.848, 8.9085) knots 0 0 0 0 1 1 1 1
  spline S232 degree 3 poles (48.848, 8.9085) (48.7512, 8.9768) (48.6658, 9.0337) (48.6573, 9.0337) knots 0 0 0 0 1 1 1 1
  spline S233 degree 3 poles (48.6573, 9.0337) (48.6516, 9.0337) (48.6174, 8.9255) (48.5861, 8.7946) knots 0 0 0 0 1 1 1 1
  spline S234 degree 3 poles (55.4945, 8.5498) (54.4641, 8.3619) (53.4678, 7.8325) (52.9042, 7.1721) knots 0 0 0 0 1 1 1 1
  spline S235 degree 3 poles (52.9042, 7.1721) (52.1898, 6.3324) (51.8368, 5.0401) (51.9336, 3.6169) knots 0 0 0 0 1 1 1 1
  spline S236 degree 3 poles (51.9336, 3.6169) (51.962, 3.1899) (52.0503, 2.521) (52.0987, 2.3644) knots 0 0 0 0 1 1 1 1
  spline S237 degree 3 poles (52.0987, 2.3644) (52.1158, 2.3132) (52.1186, 2.3132) (52.1755, 2.3673) knots 0 0 0 0 1 1 1 1
  spline S238 degree 3 poles (52.1755, 2.3673) (52.2837, 2.4669) (52.5171, 2.595) (52.6964, 2.6519) knots 0 0 0 0 1 1 1 1
  spline S239 degree 3 poles (52.6964, 2.6519) (52.964, 2.7402) (53.3369, 2.7942) (54.1026, 2.8569) knots 0 0 0 0 1 1 1 1
  spline S240 degree 3 poles (54.1026, 2.8569) (55.0903, 2.9394) (55.4917, 3.0106) (55.987, 3.1871) knots 0 0 0 0 1 1 1 1
  spline S241 degree 3 poles (55.987, 3.1871) (56.727, 3.4518) (57.487, 4.2004) (57.8884, 5.0543) knots 0 0 0 0 1 1 1 1
  spline S242 degree 3 poles (57.8884, 5.0543) (58.0279, 5.3532) (58.1588, 5.746) (58.2328, 6.0791) knots 0 0 0 0 1 1 1 1
  spline S243 degree 3 poles (58.2328, 6.0791) (58.2926, 6.3495) (58.3495, 6.8647) (58.3268, 6.9045) knots 0 0 0 0 1 1 1 1
  spline S244 degree 3 poles (58.3268, 6.9045) (58.3182, 6.9159) (58.2101, 6.8562) (58.0877, 6.7679) knots 0 0 0 0 1 1 1 1
  spline S245 degree 3 poles (58.0877, 6.7679) (57.6692, 6.4747) (56.9604, 6.1844) (56.4538, 6.099) knots 0 0 0 0 1 1 1 1
  spline S246 degree 3 poles (56.4538, 6.099) (56.3485, 6.0819) (56.1521, 6.0734) (56.0183, 6.0791) knots 0 0 0 0 1 1 1 1
  spline S247 degree 3 poles (56.0183, 6.0791) (55.7137, 6.0961) (55.6881, 6.1218) (55.7137, 6.3723) knots 0 0 0 0 1 1 1 1
  spline S248 degree 3 poles (55.7137, 6.3723) (55.7678, 6.8732) (56.0553, 7.508) (56.4139, 7.9207) knots 0 0 0 0 1 1 1 1
  spline S249 degree 3 poles (56.4139, 7.9207) (56.5477, 8.0716) (56.8352, 8.3136) (56.969, 8.3847) knots 0 0 0 0 1 1 1 1
  spline S250 degree 3 poles (56.969, 8.3847) (57.0373, 8.4217) (57.0885, 8.4616) (57.0828, 8.4786) knots 0 0 0 0 1 1 1 1
  spline S251 degree 3 poles (57.0828, 8.4786) (57.0601, 8.5413) (56.7726, 8.584) (56.2944, 8.5954) knots 0 0 0 0 1 1 1 1
  spline S252 degree 3 poles (56.2944, 8.5954) (55.8902, 8.6039) (55.7393, 8.5954) (55.4945, 8.5498) knots 0 0 0 0 1 1 1 1
  spline S253 degree 3 poles (61.1362, 7.7158) (61.0451, 7.5649) (60.9427, 7.3173) (60.8943, 7.1237) knots 0 0 0 0 1 1 1 1
  spline S254 degree 3 poles (60.8943, 7.1237) (60.7747, 6.6341) (60.7633, 6.1958) (60.8516, 5.191) knots 0 0 0 0 1 1 1 1
  spline S255 degree 3 poles (60.8516, 5.191) (60.9227, 4.3854) (60.9142, 4.3199) (60.7548, 4.3513) knots 0 0 0 0 1 1 1 1
  spline S256 degree 3 poles (60.7548, 4.3513) (60.0432, 4.4936) (59.5792, 4.9519) (59.0668, 6.0136) knots 0 0 0 0 1 1 1 1
  spline S257 degree 3 poles (59.0668, 6.0136) (58.9416, 6.2698) (58.8448, 6.4406) (58.8277, 6.4263) knots 0 0 0 0 1 1 1 1
  spline S258 degree 3 poles (58.8277, 6.4263) (58.7793, 6.3751) (58.6, 5.9026) (58.5317, 5.6407) knots 0 0 0 0 1 1 1 1
  spline S259 degree 3 poles (58.5317, 5.6407) (58.4321, 5.2621) (58.4008, 4.9889) (58.4008, 4.542) knots 0 0 0 0 1 1 1 1
  spline S260 degree 3 poles (58.4008, 4.542) (58.4008, 3.725) (58.5886, 3.0163) (58.953, 2.447) knots 0 0 0 0 1 1 1 1
  spline S261 degree 3 poles (58.953, 2.447) (59.1038, 2.2136) (59.5621, 1.7496) (59.8838, 1.5048) knots 0 0 0 0 1 1 1 1
  spline S262 degree 3 poles (59.8838, 1.5048) (60.5413, 1.0095) (61.3469, 0.6708) (62.2236, 0.5228) knots 0 0 0 0 1 1 1 1
  spline S263 degree 3 poles (62.2236, 0.5228) (62.7189, 0.4402) (62.6876, 0.4317) (62.7075, 0.6594) knots 0 0 0 0 1 1 1 1
  spline S264 degree 3 poles (62.7075, 0.6594) (62.7274, 0.9099) (62.8555, 1.3027) (63.1117, 1.9004) knots 0 0 0 0 1 1 1 1
  spline S265 degree 3 poles (63.1117, 1.9004) (63.5813, 3.002) (63.7635, 3.6368) (63.7977, 4.3029) knots 0 0 0 0 1 1 1 1
  spline S266 degree 3 poles (63.7977, 4.3029) (63.8575, 5.3817) (63.3024, 6.4605) (62.3801, 7.0668) knots 0 0 0 0 1 1 1 1
  spline S267 degree 3 poles (62.3801, 7.0668) (62.2464, 7.1579) (61.9646, 7.3201) (61.7568, 7.4283) knots 0 0 0 0 1 1 1 1
  spline S268 degree 3 poles (61.7568, 7.4283) (61.549, 7.5365) (61.3355, 7.6646) (61.2871, 7.7158) knots 0 0 0 0 1 1 1 1
  line L39 (61.2871, 7.7158) -> (61.1932, 7.8069)
  line L40 (61.1932, 7.8069) -> (61.1362, 7.7158)
extrude "Estrusione4" cut sketch "Schizzo3" against normal blind 6 contours S0 S1 S2 S3 S4 S5 S6 S7 S8 S9 S10 S11 S12 S13 S14 S15 S16 S17 S18 S19 L9 L10 | S20 S21 S22 S23 L11 L12 S24 L13 L14 S25 S26 S27 S28 S29 S30 S31 S32 S33 S34 S35 | S36 S37 S38 S39 S40 S41 S42 S43 S44 S45 S46 S47 S48 S49 S50 S51 S52 S53 S54 S55 S56 | S57 S58 S59 S60 S61 S62 S63 S64 S65 S66 S67 L15 L16 S68 S69 S70 S71 S72 L17 L18 S73 S74 S75 | S76 S77 S78 S79 S80 S81 S82 L19 L20 S83 S84 S85 L21 L22 S86 S87 L23 L24 S88 S89 S90 S91 | S92 S93 S94 S95 S96 S97 S98 | S99 L25 L26 S100 S101 S102 S103 S104 S105 S106 S107 L27 L28 S108 S109 S110 S111 S112 S113 S114 S115 | S116 S117 S118 S119 S120 L29 L30 S121 S122 S123 S124 S125 S126 S127 S128 S129 S130 S131 | S132 S133 S134 S135 S136 S137 S138 S139 S140 S141 L31 L32 S142 S143 S144 S145 S146 S147 S148 S149 | S150 S151 S152 S153 S154 S155 S156 S157 S158 S159 S160 S161 S162 S163 L33 L34 S164 S165 | S166 S167 S168 S169 S170 | S171 S172 S173 S174 S175 S176 S177 S178 S179 S180 S181 S182 S183 S184 L35 L36 S185 S186 S187 S188 | S189 S190 S191 S192 S193 S194 S195 S196 S197 S198 S199 S200 S201 S202 S203 S204 S205 S206 S207 S208 S209 | S210 S211 S212 S213 S214 | S215 S216 S217 S218 L37 L38 S219 S220 S221 S222 S223 S224 S225 S226 S227 S228 S229 S230 S231 S232 S233 | S234 S235 S236 S237 S238 S239 S240 S241 S242 S243 S244 S245 S246 S247 S248 S249 S250 S251 S252 | S253 S254 S255 S256 S257 S258 S259 S260 S261 S262 S263 S264 S265 S266 S267 S268 L39 L40
sketch "Schizzo2" plane through (0, 0, 0) normal (0, -1, 0) x (1, 0, 0)
  arc A0 (30.3523, 1.6578) -> (32.4515, -2.2) centre (32.4515, 0.3) ccw
  line L0 (32.4515, -2.2) -> (81.6844, -2.2)
  arc A1 (81.6844, -2.2) -> (84.16, -0.0479) centre (81.6844, 0.3) ccw
  line L1 (84.16, -0.0479) -> (84.7152, 3.9025)
  arc A2 (84.7152, 3.9025) -> (84.0769, 4.7495) centre (83.9725, 4.0068) ccw
  line L2 (84.0769, 4.7495) -> (83.3837, 4.847)
  arc A3 (83.3837, 4.847) -> (82.5366, 4.2086) centre (83.2793, 4.1043) ccw
  line L3 (82.5366, 4.2086) -> (81.9451, 0)
  line L4 (81.9451, 0) -> (79.5451, 0)
  line L5 (79.5451, 0) -> (59.0337, 76.5496)
  arc A4 (59.0337, 76.5496) -> (58.1152, 77.08) centre (58.3093, 76.3555) ccw
  line L6 (58.1152, 77.08) -> (57.439, 76.8988)
  arc A5 (57.439, 76.8988) -> (56.9087, 75.9802) centre (57.6331, 76.1743) ccw
  line L7 (56.9087, 75.9802) -> (60.9123, 61.0387)
  arc A6 (58.387, 45.0001) -> (60.9123, 61.0387) centre (41.5938, 55.8623) ccw
  line L8 (58.387, 45.0001) -> (30.3523, 1.6578)
  line L9 (64.4935, 30.009) -> (67.3802, 35.009)
  line L10 (67.3802, 35.009) -> (64.4935, 40.009)
  line L11 (64.4935, 40.009) -> (58.72, 40.009)
  line L12 (58.72, 40.009) -> (55.8332, 35.009)
  line L13 (55.8332, 35.009) -> (58.72, 30.009)
  line L14 (58.72, 30.009) -> (64.4935, 30.009)
  line L15 (68.4935, 16.009) -> (71.3802, 21.009)
  line L16 (71.3802, 21.009) -> (68.4935, 26.009)
  line L17 (68.4935, 26.009) -> (62.72, 26.009)
  line L18 (62.72, 26.009) -> (59.8332, 21.009)
  line L19 (62.72, 16.009) -> (68.4935, 16.009)
  line L20 (59.8332, 21.009) -> (62.72, 16.009)
  line L21 (58.72, 2.009) -> (64.4935, 2.009)
  line L22 (64.4935, 2.009) -> (67.3802, 7.009)
  line L23 (67.3802, 7.009) -> (64.4935, 12.009)
  line L24 (64.4935, 12.009) -> (58.72, 12.009)
  line L25 (58.72, 12.009) -> (55.8332, 7.009)
  line L26 (55.8332, 7.009) -> (58.72, 2.009)
  line L27 (54.4935, 16.009) -> (57.3802, 21.009)
  line L28 (57.3802, 21.009) -> (54.4935, 26.009)
  line L29 (54.4935, 26.009) -> (48.72, 26.009)
  line L30 (48.72, 26.009) -> (45.8332, 21.009)
  line L31 (45.8332, 21.009) -> (48.72, 16.009)
  line L32 (48.72, 16.009) -> (54.4935, 16.009)
  line L33 (50.4935, 2.009) -> (53.3802, 7.009)
  line L34 (53.3802, 7.009) -> (50.4935, 12.009)
  line L35 (50.4935, 12.009) -> (44.72, 12.009)
  line L36 (44.72, 12.009) -> (41.8332, 7.009)
  line L37 (44.72, 2.009) -> (50.4935, 2.009)
  line L38 (41.8332, 7.009) -> (44.72, 2.009)
  point P0 (61.6067, 35.009)
  dimension "d24" = 5
  constraint horizontal L11
  constraint horizontal L17
  constraint horizontal L24
  constraint horizontal L29
  constraint horizontal L35
  measures "d24" distance of P0 L14
extrude "Estrusione3" [rolled back] along distance -9 taper angle 0
